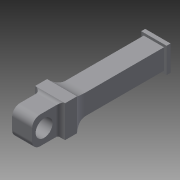
# Autodesk Inventor part: arm-seg2
Saved by Autodesk Inventor 2016 (Build 200138000, 138)
## iProperties
Created: 2015-10-13
Part Number: arm-seg2
Material: Generic
Document SubType Name: Modeling
Designer: eedoga
Density: 1 g/cm^3
Appearance: Default
Author: eedoga
Autodesk Inventor part; units mm, degrees
ref_plane "YZ Plane" through (0, 0, 0) normal (1, 0, 0) x (0, 1, 0)
ref_plane "XZ Plane" through (0, 0, 0) normal (0, 1, 0) x (-1, 0, 0)
ref_plane "XY Plane" through (0, 0, 0) normal (0, 0, 1) x (1, 0, 0)
sketch "Sketch1" plane through (0, 0, 0) normal (0, 0, 1) x (1, 0, 0)
  line L0 (-3.175, -3.175) -> (-3.175, 3.175) projected
  line L1 (-3.175, 3.175) -> (3.175, 3.175) projected
  line L2 (3.175, 3.175) -> (3.175, -3.175) projected
  line L3 (3.175, -3.175) -> (-3.175, -3.175) projected
  line L4 (-5, -5) -> (5, -5) projected
  line L5 (5, -5) -> (5, 5) projected
  line L6 (5, 5) -> (-5, 5) projected
  line L7 (-5, 5) -> (-5, -5) projected
  line L8 (-4.1303, 4.1303) -> (4.1303, 4.1303) projected
  line L9 (4.1303, 4.1303) -> (4.1303, -4.1303) projected
  line L10 (-4.1303, -4.1303) -> (-4.1303, 4.1303) projected
  line L11 (4.1303, -4.1303) -> (-4.1303, -4.1303) projected
  line L12 (2.54, -2.54) -> (-2.54, -2.54)
  line L13 (-2.54, -2.54) -> (-2.54, 2.54)
  line L14 (-2.54, 2.54) -> (2.54, 2.54)
  line L15 (2.54, 2.54) -> (2.54, -2.54)
  line L16 (2.54, -2.54) -> (-2.54, 2.54) construction
  line L17 (-2.54, -2.54) -> (2.54, 2.54) construction
  point P0 (0, 0)
  dimension "d0" = 5.08
  dimension "d1" = 5.08
  constraints: 12 end point, 2 midpoint, 2 parallel, 1 horizontal, 1 perpendicular
  measures "d0" distance of L13.end L14.end
  measures "d1" distance of L12.end L13.end
extrude "Extrusion1" add sketch "Sketch1" along normal blind 25 contours L12 L13 L14 L15
sketch "Sketch2" plane through (0, 0, 0) normal (0, 0, -1) x (-1, 0, 0)
  line L0 (-3.175, -3.175) -> (-3.175, 3.175) projected
  line L1 (3.175, 3.175) -> (3.175, -3.175) projected
  line L2 (-3.175, -3.175) -> (3.175, -3.175)
  line L3 (3.175, -3.175) -> (3.175, 3.175)
  line L4 (3.175, 3.175) -> (-3.175, 3.175)
  line L5 (-3.175, 3.175) -> (-3.175, -3.175)
  point P0 (0, 0)
  constraints: 8 end point, 2 parallel, 1 horizontal, 1 perpendicular
extrude "Extrusion2" add sketch "Sketch2" along normal blind 1
sketch "Sketch3" plane through (0, 0, 25) normal (0, 0, 1) x (1, 0, 0)
  line L0 (3.75, -4) -> (-3.75, -4)
  line L1 (-3.75, -4) -> (-3.75, 4)
  line L2 (-3.75, 4) -> (3.75, 4)
  line L3 (3.75, 4) -> (3.75, -4)
  line L4 (3.75, -4) -> (-3.75, 4) construction
  line L5 (-3.75, -4) -> (3.75, 4) construction
  point P0 (0, 0)
  dimension "d6" = 7.5
  dimension "d7" = 8
  constraints: 12 end point, 2 midpoint, 2 parallel, 1 horizontal, 1 perpendicular
  measures "d6" distance of L1.end L2.end
  measures "d7" distance of L0.end L1.end
extrude "Extrusion3" add sketch "Sketch3" along normal blind 1 and the other way blind 2
fillet "Fillet1" radius 5 4 edges at (0, 2.54, 23) (2.54, 0, 23) (-2.54, 0, 23) (0, -2.54, 23)
sketch "Sketch4" plane through (0, 0, 26) normal (0, 0, 1) x (1, 0, 0)
  line L0 (2.5088, -3.4457) -> (-2.5088, -3.4457)
  line L1 (-2.5088, -3.4457) -> (-2.5088, 3.4457)
  line L2 (-2.5088, 3.4457) -> (2.5088, 3.4457)
  line L3 (2.5088, 3.4457) -> (2.5088, -3.4457)
  line L4 (2.5088, -3.4457) -> (-2.5088, 3.4457) construction
  line L5 (-2.5088, -3.4457) -> (2.5088, 3.4457) construction
  point P0 (0, 0)
  constraints: 12 end point, 2 midpoint, 2 parallel, 1 horizontal, 1 perpendicular
extrude "Extrusion4" add sketch "Sketch4" along normal blind 7
sketch "Sketch5" plane through (-2.5088, -3.4457, 26) normal (-1, 0, 0) x (0, 0, 1)
  line L0 (0, 6.8913) -> (7, 6.8913) projected
  line L1 (0, 0) -> (4, 0)
  line L2 (4, 0) -> (4, 6.8913)
  line L3 (4, 6.8913) -> (0, 6.8913)
  line L4 (0, 6.8913) -> (0, 0)
  circle A0 centre (4, 3.4457) radius 2.125
  point P0 (-26, 3.4457)
  dimension "d15" = 4
  dimension "d16" = 4.25
  constraints: 8 end point, 2 parallel, 1 centre point, 1 horizontal, 1 midpoint, 1 perpendicular, 1 point on line
  measures "d15" distance of L3.end L2.end
  measures "d16" diameter of A0
extrude "Extrusion5" cut sketch "Sketch5" against normal blind 7 contours A0 L2 | L2 A0
fillet "Fillet2" radius 1 4 edges at (-2.5088, 0, 26) (0, -3.4457, 26) (2.5088, 0, 26) (0, 3.4457, 26)
fillet "Fillet3" radius 2 2 edges at (0, -3.4457, 33) (0, 3.4457, 33)
body "Solid1"
